Autodesk Inventor part; units mm, degrees
(part 2 of 2)
sketch "Эскиз10" plane through (-610.2675, -276.6936, 281.5883) normal (-1, 0, 0) x (0, 0, 1)
  line L0 (146.75, 43.7049) -> (146.75, 61.7049) projected
  line L1 (141.75, 51.2049) -> (148.25, 51.2049) projected
  line L2 (148.25, 51.2049) -> (148.25, 54.2049) projected
  line L3 (148.25, 54.2049) -> (141.75, 54.2049) projected
  line L4 (143.25, 61.7049) -> (143.25, 43.7049) projected
  line L5 (146.75, 61.7049) -> (143.25, 61.7049) projected
  line L6 (141.75, 54.2049) -> (141.75, 51.2049) projected
  line L7 (143.25, 43.7049) -> (146.75, 43.7049) projected
  line L8 (106.125, 43.7049) -> (109.625, 43.7049) projected
  line L9 (195, 59.705) -> (195, -6.7721) projected
  line L10 (187, 59.705) -> (195, 59.705) projected
  line L11 (187, 59.705) -> (187, 55.705) projected
  line L12 (187, 55.705) -> (175, 55.705) projected
  line L13 (175, 55.705) -> (175, 59.705) projected
  line L14 (175, 59.705) -> (175, 60.705) projected
  line L15 (175, 60.705) -> (155, 60.705) projected
  line L16 (155, 60.705) -> (155, 59.705) projected
  line L17 (155, 59.705) -> (155, 55.705) projected
  line L18 (155, 55.705) -> (135, 55.705) projected
  line L19 (135, 55.705) -> (135, 59.705) projected
  line L20 (135, 59.705) -> (135, 60.705) projected
  line L21 (135, 60.705) -> (115, 60.705) projected
  line L22 (115, 60.705) -> (115, 59.705) projected
  line L23 (115, 59.705) -> (115, 55.705) projected
  line L24 (115, 55.705) -> (80, 55.705) projected
  line L25 (80, 55.705) -> (80, 59.705) projected
  line L26 (80, 59.705) -> (80, 60.705) projected
  line L27 (80, 60.705) -> (60, 60.705) projected
  line L28 (60, 60.705) -> (60, 59.705) projected
  line L29 (60, 59.705) -> (60, 55.705) projected
  line L30 (60, 55.705) -> (40, 55.705) projected
  line L31 (40, 55.705) -> (40, 59.705) projected
  line L32 (40, 59.705) -> (40, 60.705) projected
  line L33 (40, 60.705) -> (20, 60.705) projected
  line L34 (20, 60.705) -> (20, 59.705) projected
  line L35 (20, 59.705) -> (20, 55.705) projected
  line L36 (20, 55.705) -> (8, 55.705) projected
  line L37 (8, 55.705) -> (8, 59.705) projected
  line L38 (0, 59.705) -> (8, 59.705) projected
  line L39 (0, 59.705) -> (0, -6.7721) projected
  line L40 (37.2102, 33.4561) -> (37.2102, 26.5911) projected
  line L41 (37.2102, 26.5911) -> (39.3474, 26.5911) projected
  line L42 (39.3474, 26.5911) -> (39.3474, 33.4561) projected
  line L43 (40.5317, 33.4561) -> (40.5317, 25.9989) projected
  line L44 (39.9395, 25.416) -> (34.5456, 25.416) projected
  line L45 (32.7044, 27.2387) -> (32.7044, 33.4561) projected
  line L46 (33.8887, 33.4561) -> (33.8887, 27.248) projected
  line L47 (34.5456, 26.5911) -> (36.0259, 26.5911) projected
  line L48 (36.0259, 26.5911) -> (36.0259, 33.4561) projected
  line L49 (42.5949, 30.3197) -> (46.1292, 30.3197) projected
  line L50 (46.1292, 30.3197) -> (46.1292, 32.2164) projected
  line L51 (45.4908, 32.8733) -> (42.5949, 32.8733) projected
  line L52 (42.5949, 34.0483) -> (45.4908, 34.0483) projected
  line L53 (47.3135, 32.2164) -> (47.3135, 27.2387) projected
  line L54 (45.4908, 25.416) -> (43.8254, 25.416) projected
  line L55 (41.9935, 27.248) -> (41.9935, 29.7275) projected
  line L56 (62.3389, 25.9989) -> (62.3389, 33.4561) projected
  line L57 (62.9311, 34.0483) -> (65.827, 34.0483) projected
  line L58 (67.6589, 32.2164) -> (67.6589, 25.9989) projected
  line L59 (66.4746, 25.9989) -> (66.4746, 32.2071) projected
  line L60 (65.827, 32.8733) -> (63.5232, 32.8733) projected
  line L61 (63.5232, 32.8733) -> (63.5232, 25.9989) projected
  line L62 (70.9434, 34.0575) -> (73.2564, 34.0575) projected
  line L63 (73.2564, 34.0575) -> (73.2564, 36.7776) projected
  line L64 (74.4407, 36.7776) -> (74.4407, 25.9989) projected
  line L65 (73.8486, 25.416) -> (70.9434, 25.416) projected
  line L66 (69.1207, 27.2295) -> (69.1207, 32.2164) projected
  line L67 (75.9025, 27.2387) -> (75.9025, 32.2164) projected
  line L68 (77.7437, 34.0483) -> (79.3813, 34.0483) projected
  line L69 (81.2225, 32.2164) -> (81.2225, 27.2387) projected
  line L70 (79.3813, 25.416) -> (78.4284, 25.416) projected
  line L71 (78.4284, 25.416) -> (80.9172, 23.1493) projected
  line L72 (80.6304, 22.0945) -> (76.4947, 22.0945) projected
  line L73 (76.4947, 23.2696) -> (79.4369, 23.2696) projected
  line L74 (79.4369, 23.2696) -> (76.3651, 26.0729) projected
  line L75 (84.6088, 34.0483) -> (86.2649, 34.0483) projected
  line L76 (88.0968, 32.2164) -> (88.0968, 27.2387) projected
  line L77 (86.2649, 25.416) -> (83.369, 25.416) projected
  line L78 (82.7769, 25.9989) -> (82.7769, 32.2349) projected
  line L79 (103.1778, 23.2696) -> (104.8154, 23.2696) projected
  line L80 (104.8154, 22.0945) -> (103.1778, 22.0945) projected
  line L81 (109.7838, 30.9673) -> (109.7838, 32.2164) projected
  line L82 (111.625, 34.0483) -> (113.6975, 34.0483) projected
  line L83 (114.2896, 33.4561) -> (114.2896, 25.9989) projected
  line L84 (113.1053, 25.9989) -> (113.1053, 29.1446) projected
  line L85 (113.1053, 29.1446) -> (111.6157, 29.1446) projected
  line L86 (131.9611, 29.1446) -> (129.3891, 33.1508) projected
  line L87 (130.4068, 33.6412) -> (132.7383, 29.9403) projected
  line L88 (133.4415, 30.8378) -> (133.4415, 33.4561) projected
  line L89 (134.6258, 33.4561) -> (134.6258, 25.9989) projected
  line L90 (133.4415, 25.9989) -> (133.4415, 29.3482) projected
  line L91 (133.4415, 29.3482) -> (130.3605, 25.7121) projected
  line L92 (142.8694, 25.9989) -> (142.8694, 33.4561) projected
  line L93 (143.4615, 34.0483) -> (146.3574, 34.0483) projected
  line L94 (148.1894, 32.2164) -> (148.1894, 25.9989) projected
  line L95 (147.0051, 25.9989) -> (147.0051, 32.2071) projected
  line L96 (146.3574, 32.8733) -> (144.0537, 32.8733) projected
  line L97 (144.0537, 32.8733) -> (144.0537, 25.9989) projected
  line L98 (156.433, 24.7499) -> (156.433, 31.3837) projected
  line L99 (159.1069, 34.0483) -> (159.9303, 34.0483) projected
  line L100 (162.5949, 31.3837) -> (162.5949, 24.7499) projected
  line L101 (159.9303, 22.0945) -> (159.1069, 22.0945) projected
  line L102 (149.6419, 25.9989) -> (149.6419, 33.4561) projected
  line L103 (150.8262, 33.4561) -> (150.8262, 26.5911) projected
  line L104 (150.8262, 26.5911) -> (152.251, 26.5911) projected
  line L105 (152.251, 26.5911) -> (153.8239, 33.6504) projected
  line L106 (154.9619, 33.3451) -> (153.2873, 25.8046) projected
  line L107 (152.7229, 25.416) -> (150.2341, 25.416) projected
  line L108 (136.0783, 27.2387) -> (136.0783, 32.2164) projected
  line L109 (137.9288, 34.0483) -> (139.5664, 34.0483) projected
  line L110 (141.4168, 32.2164) -> (141.4168, 23.9172) projected
  line L111 (138.8817, 25.416) -> (137.9288, 25.416) projected
  line L112 (122.524, 27.2387) -> (122.524, 32.2164) projected
  line L113 (124.3559, 34.0483) -> (126.012, 34.0483) projected
  line L114 (127.8439, 32.2164) -> (127.8439, 27.2387) projected
  line L115 (126.012, 25.416) -> (124.3559, 25.416) projected
  line L116 (115.7329, 27.2387) -> (115.7329, 32.2164) projected
  line L117 (117.5833, 34.0483) -> (119.221, 34.0483) projected
  line L118 (121.0714, 32.2164) -> (121.0714, 23.9172) projected
  line L119 (118.5363, 25.416) -> (117.5833, 25.416) projected
  line L120 (108.1277, 25.9989) -> (108.1277, 33.4561) projected
  line L121 (109.312, 33.4561) -> (109.312, 25.9989) projected
  line L122 (101.3366, 25.9897) -> (101.3366, 33.4561) projected
  line L123 (101.9288, 34.0483) -> (104.8247, 34.0483) projected
  line L124 (106.6566, 32.2071) -> (106.6566, 25.9897) projected
  line L125 (105.4723, 25.9897) -> (105.4723, 32.2071) projected
  line L126 (104.8247, 32.8733) -> (102.5209, 32.8733) projected
  line L127 (102.5209, 32.8733) -> (102.5209, 25.9897) projected
  line L128 (92.1215, 29.1446) -> (89.5494, 33.1508) projected
  line L129 (90.5672, 33.6412) -> (92.8987, 29.9403) projected
  line L130 (93.6018, 30.8378) -> (93.6018, 33.4561) projected
  line L131 (94.7861, 33.4561) -> (94.7861, 25.9989) projected
  line L132 (93.6018, 25.9989) -> (93.6018, 29.3482) projected
  line L133 (93.6018, 29.3482) -> (90.5209, 25.7121) projected
  line L134 (55.5571, 27.2387) -> (55.5571, 32.2164) projected
  line L135 (57.389, 34.0483) -> (59.0452, 34.0483) projected
  line L136 (60.8771, 32.2164) -> (60.8771, 27.2387) projected
  line L137 (59.0452, 25.416) -> (57.389, 25.416) projected
  line L138 (48.7661, 25.9989) -> (48.7661, 33.4561) projected
  line L139 (49.9503, 33.4561) -> (49.9503, 26.5911) projected
  line L140 (49.9503, 26.5911) -> (51.3752, 26.5911) projected
  line L141 (51.3752, 26.5911) -> (52.948, 33.6504) projected
  line L142 (54.086, 33.3451) -> (52.4114, 25.8046) projected
  line L143 (51.847, 25.416) -> (49.3582, 25.416) projected
  line L144 (111.125, 51.2049) -> (111.125, 54.2049) projected
  line L145 (104.625, 51.2049) -> (111.125, 51.2049) projected
  line L146 (109.625, 49.7049) -> (109.625, 55.7049) projected
  line L147 (111.125, 54.2049) -> (104.625, 54.2049) projected
  line L148 (109.625, 55.7049) -> (106.125, 55.7049) projected
  line L149 (106.125, 55.7049) -> (106.125, 49.7049) projected
  line L150 (104.625, 54.2049) -> (104.625, 51.2049) projected
  line L151 (106.125, 49.7049) -> (106.125, 43.7049) projected
  line L152 (109.625, 43.7049) -> (109.625, 49.7049) projected
  line L153 (90.3751, 51.2049) -> (90.3751, 54.2049) projected
  line L154 (83.8751, 51.2049) -> (90.3751, 51.2049) projected
  line L155 (90.3751, 54.2049) -> (83.8751, 54.2049) projected
  line L156 (88.8751, 49.7049) -> (88.8751, 55.7049) projected
  line L157 (88.8751, 55.7049) -> (85.3751, 55.7049) projected
  line L158 (85.3751, 55.7049) -> (85.3751, 49.7049) projected
  line L159 (83.8751, 54.2049) -> (83.8751, 51.2049) projected
  line L160 (85.3751, 49.7049) -> (85.3751, 43.7049) projected
  line L161 (88.8751, 43.7049) -> (88.8751, 49.7049) projected
  line L162 (85.3751, 43.7049) -> (88.8751, 43.7049) projected
  line L163 (48.25, 43.7049) -> (51.75, 43.7049) projected
  line L164 (51.75, 43.7049) -> (51.75, 61.7049) projected
  line L165 (53.25, 51.2049) -> (53.25, 54.2049) projected
  line L166 (46.75, 51.2049) -> (53.25, 51.2049) projected
  line L167 (53.25, 54.2049) -> (46.75, 54.2049) projected
  line L168 (46.75, 54.2049) -> (46.75, 51.2049) projected
  line L169 (51.75, 61.7049) -> (48.25, 61.7049) projected
  line L170 (48.25, 61.7049) -> (48.25, 43.7049) projected
  line L171 (175, -6.7721) -> (195, -6.7721) projected
  line L172 (20, -6.7721) -> (20, -10.7721) projected
  line L173 (20, -10.7721) -> (40, -10.7721) projected
  line L174 (40, -10.7721) -> (40, -6.7721) projected
  line L175 (60, -6.7721) -> (60, -10.7721) projected
  line L176 (60, -10.7721) -> (80, -10.7721) projected
  line L177 (80, -10.7721) -> (80, -6.7721) projected
  line L178 (115, -6.7721) -> (115, -10.7721) projected
  line L179 (115, -10.7721) -> (135, -10.7721) projected
  line L180 (135, -10.7721) -> (135, -6.7721) projected
  line L181 (155, -6.7721) -> (155, -10.7721) projected
  line L182 (155, -10.7721) -> (175, -10.7721) projected
  line L183 (175, -10.7721) -> (175, -6.7721) projected
  line L184 (0, -6.7721) -> (20, -6.7721) projected
  line L185 (40, -6.7721) -> (60, -6.7721) projected
  line L186 (80, -6.7721) -> (115, -6.7721) projected
  line L187 (135, -6.7721) -> (155, -6.7721) projected
  point P0 (-281.5883, 276.6936)
  point P1 (48.25, 51.2049)
  point P2 (51.75, 51.2049)
  point P3 (51.75, 54.2049)
  point P4 (48.25, 54.2049)
  point P5 (85.3751, 54.2049)
  point P6 (85.3751, 51.2049)
  point P7 (88.8751, 51.2049)
  point P8 (88.8751, 54.2049)
  point P9 (109.625, 51.2049)
  point P10 (109.625, 54.2049)
  point P11 (106.125, 54.2049)
  point P12 (106.125, 51.2049)
  point P13 (146.75, 51.2049)
  point P14 (146.75, 54.2049)
  point P15 (143.25, 54.2049)
  point P16 (143.25, 51.2049)
  point P17 (51.75, 55.705)
  point P18 (48.25, 55.705)
  constraints: 139 other
extrude "Выдавливание12" cut sketch "Эскиз10" against normal blind 6 contours L7 L4 L1 L0 | L1 L4 L3 L0 | L0 L3 L2 L1 | L3 L4 L18 L0 | L1 L6 L3 L4 | L18 L4 L5 L0 | L146 L147 L149 L24 | L147 L144 L145 L146 | L146 L145 L149 L147 | L156 L155 L158 L24 | L149 L145 L150 L147 | L146 L152 L8 L151 L149 L145 | L156 L154 L158 L155 | L155 L153 L154 L156 | L158 L154 L159 L155 | L164 L167 L170 L30 | L167 L165 L166 L164 | L164 L166 L170 L167 | L170 L166 L168 L167 | L164 L163 L170 L166
extrude "Выдавливание13" cut sketch "Эскиз6" against normal blind 6 contours L60 L70 L71 L68 | L60 L66 L71 L70 | L71 L70 L61 L68 | L68 L61 L65 L71 | L71 L66 L61 L70 | L61 L70 L67 L68 | L71 L64 L61 L66 | L61 L66 L67 L70 | L72 L85 L79 L75 | L72 L73 L79 L85 | L79 L85 L80 L75 | L79 L73 L80 L85 | L80 L85 L81 L75 | L79 L84 L81 L73 | L80 L73 L81 L85 | L81 L85 L74 L75 | L81 L73 L74 L85 | L86 L92 L97 L87 | L92 L95 L96 L94 L89 L86 | L86 L89 L97 L92 | L97 L92 L98 L87 | L86 L88 L97 L89 | L97 L89 L98 L92 | L97 L88 L98 L89 | L98 L89 L90 L92 | L99 L102 L108 L109 | L102 L101 L105 L99 | L99 L105 L108 L102 | L108 L102 L107 L109 | L99 L100 L108 L105 | L108 L105 L107 L102 | L108 L100 L107 L105 | L107 L105 L106 L102
sketch "Эскиз14" plane through (-610.2675, -276.6936, 281.5883) normal (-1, 0, 0) x (0, 0, 1)
  line L0 (88.8751, 55.7049) -> (85.3751, 55.7049) projected
  line L1 (88.8751, 55.7049) -> (85.3751, 55.7049)
  line L2 (85.3751, 55.7049) -> (85.3751, 43.5901)
  line L3 (85.3751, 43.5901) -> (88.8751, 43.5901)
  line L4 (88.8751, 43.5901) -> (88.8751, 55.7049)
  line L5 (88.8751, -6.7722) -> (85.3751, -6.7722)
  line L6 (85.3751, -6.7722) -> (85.3751, 5.3427)
  line L7 (85.3751, 5.3427) -> (88.8751, 5.3427)
  line L8 (88.8751, 5.3427) -> (88.8751, -6.7722)
  point P0 (-281.5883, 276.6936)
  point P1 (85.3751, 55.7049)
  dimension "d66" = 3.5
  constraints: 16 end point, 4 parallel, 2 horizontal, 2 perpendicular, 1 collinear
  measures "d66" distance of L2.end L3.end
extrude "Выдавливание14" cut sketch "Эскиз14" against normal blind 6
sketch "Эскиз15" plane through (-610.2675, -276.6936, 281.5883) normal (-1, 0, 0) x (0, 0, 1)
  line L0 (106.125, -5.263) -> (106.125, -6.763) projected
  line L1 (106.125, -5.263) -> (109.625, -5.263)
  line L2 (109.625, -5.263) -> (109.625, -7.3348)
  line L3 (109.625, -7.3348) -> (106.125, -7.3348)
  line L4 (106.125, -7.3348) -> (106.125, -5.263)
  line L5 (88.8751, 54.2049) -> (85.3751, 54.2049)
  line L6 (85.3751, 54.2049) -> (85.3751, 56.0756)
  line L7 (85.3751, 56.0756) -> (88.8751, 56.0756)
  line L8 (88.8751, 56.0756) -> (88.8751, 54.2049)
  line L9 (109.625, 54.2049) -> (106.125, 54.2049)
  line L10 (106.125, 54.2049) -> (106.125, 56.3003)
  line L11 (106.125, 56.3003) -> (109.625, 56.3003)
  line L12 (109.625, 56.3003) -> (109.625, 54.2049)
  point P0 (-281.5883, 276.6936)
  constraints: 24 end point, 6 parallel, 3 horizontal, 3 perpendicular, 1 point on line
extrude "Выдавливание15" cut sketch "Эскиз15" against normal blind 6
